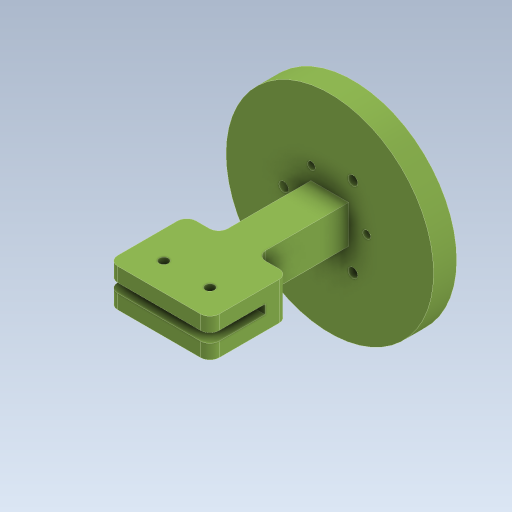
# Autodesk Inventor part: WTS_RW_base
Saved by Autodesk Inventor 2023 (Build 270158000, 158)
## iProperties
Created: 2023-05-16
Part Number: WTS_RW_base
Material: Generic
Document SubType Name: Modeling
Designer: adars
Density: 1 g/cm^3
Appearance: Olive Green
Author: adars
Autodesk Inventor part; units mm, degrees
ref_plane "YZ Plane" through (0, 0, 0) normal (1, 0, 0) x (0, 1, 0)
ref_plane "XZ Plane" through (0, 0, 0) normal (0, 1, 0) x (-1, 0, 0)
ref_plane "XY Plane" through (0, 0, 0) normal (0, 0, 1) x (1, 0, 0)
sketch "Sketch1" plane through (0, 0, 0) normal (0, 0, 1) x (1, 0, 0)
  circle A0 centre (0, 0) radius 22.5
  circle A1 centre (-10, 0) radius 1.05
  circle A2 centre (8, 0) radius 0.85
  circle A3 centre (5, -8.6603) radius 1.05
  circle A4 centre (5, 8.6603) radius 1.05
  circle A5 centre (-4, 6.9282) radius 0.85
  circle A6 centre (-4, -6.9282) radius 0.85
  dimension "d0" = 45
  dimension "d1" = 1.7
  dimension "d2" = 2.1
  dimension "d3" = 10
  dimension "d4" = 8
  dimension "d7" = 360
  dimension "d11" = 360
  constraints: 7 centre point, 2 horizontal alignment, 1 coincident, 14 other
  measures "d0" diameter of A0
  measures "d1" diameter of A2
  measures "d2" diameter of A1
  measures "d3" distance of point (0, 0) A1.centre
  measures "d4" distance of point (0, 0) A2.centre
extrude "Extrusion1" add sketch "Sketch1" along normal blind 5
sketch "Sketch2" plane through (0, 0, 5) normal (0, 0, 1) x (1, 0, 0)
  line L0 (-4.1, -4.1) -> (4.1, -4.1)
  line L1 (4.1, -4.1) -> (4.1, 4.1)
  line L2 (4.1, 4.1) -> (-4.1, 4.1)
  line L3 (-4.1, 4.1) -> (-4.1, -4.1)
  line L4 (-4.1, -4.1) -> (4.1, 4.1) construction
  line L5 (4.1, -4.1) -> (-4.1, 4.1) construction
  point P0 (0, 0)
  dimension "d15" = 8.2
  dimension "d16" = 8.2
  constraints: 12 end point, 2 midpoint, 2 parallel, 1 horizontal, 1 perpendicular
  measures "d15" distance of L2.end L1.end
  measures "d16" distance of L1.end L0.end
extrude "Extrusion2" cut sketch "Sketch2" against normal blind 3
sketch "Sketch3" plane through (0, 0, 5) normal (0, 0, 1) x (1, 0, 0)
  line L0 (4.1, 4.1) -> (4.1, -4.1) projected
  line L1 (-4.1, 4.1) -> (4.1, 4.1) projected
  line L2 (-4.1, -4.1) -> (-4.1, 4.1) projected
  line L3 (4.1, -4.1) -> (-4.1, -4.1) projected
  point P0 (0, 0)
extrude "Extrusion3" add sketch "Sketch3" along normal blind 20 and the other way blind 3
sketch "Sketch4" plane through (0, 0, 25) normal (0, 0, 1) x (1, 0, 0)
  line L0 (-11, 4.1) -> (11, 4.1)
  line L1 (11, 4.1) -> (11, -4.1)
  line L2 (11, -4.1) -> (-11, -4.1)
  line L3 (-11, -4.1) -> (-11, 4.1)
  line L4 (-11, 4.1) -> (11, -4.1) construction
  line L5 (11, 4.1) -> (-11, -4.1) construction
  point P0 (0, 0)
  dimension "d23" = 22
  dimension "d24" = 8.2
  constraints: 12 end point, 2 midpoint, 2 parallel, 1 horizontal, 1 perpendicular
  measures "d23" distance of L1.end L2.end
  measures "d24" distance of L0.end L1.end
extrude "Extrusion4" add sketch "Sketch4" along normal blind 17
sketch "Sketch5" plane through (0, 0, 42) normal (0, 0, 1) x (1, 0, 0)
  line L0 (11, -4.1) -> (11, 4.1) projected
  line L1 (-11, 1) -> (11, 1)
  line L2 (11, 1) -> (11, -1)
  line L3 (11, -1) -> (-11, -1)
  line L4 (-11, -1) -> (-11, 1)
  line L5 (-11, 1) -> (11, -1) construction
  line L6 (11, 1) -> (-11, -1) construction
  point P0 (0, 0)
  dimension "d27" = 2
  constraints: 12 end point, 2 midpoint, 2 parallel, 1 horizontal, 1 perpendicular, 1 point on line
  measures "d27" distance of L1.end L2.end
extrude "Extrusion5" cut sketch "Sketch5" against normal blind 12
sketch "Sketch6" plane through (-4.1, 4.1, 5) normal (0, 1, 0) x (1, 0, 0)
  circle A0 centre (-0.9, -31) radius 1
  line L0 (-6.9, -20) -> (-6.9, -37) projected
  line L1 (15.1, -37) -> (-6.9, -37) projected
  point P0 (4.1, 5)
  dimension "d30" = 6
  dimension "d31" = 6
  dimension "d32" = 2
  constraints: 1 centre point
  measures "d30" distance from line of L0 A0.centre
  measures "d31" distance from line of L1 A0.centre
  measures "d32" diameter of A0
extrude "Extrusion6" cut sketch "Sketch6" against normal through all
mirror "Mirror1" about plane through (0, 0, 0) normal (1, 0, 0) of "Extrusion6"
fillet "Fillet1" radius 2 8 edges at (11, 2.55, 42) (11, -2.55, 42) (11, 0, 25) (4.1, 0, 25) (-4.1, 0, 25) (-11, 0, 25) (-11, -2.55, 42) (-11, 2.55, 42)
body "Solid1"
